# Autodesk Inventor part: Grooved Pulley2
Saved by Autodesk Inventor 2014 (Build 180170000, 170)
## iProperties
Created: 2017-06-15
Part Number: Grooved Pulley2
Material: Steel
Document SubType Name: Modeling
Designer: RMcComber
Density: 1 g/cm^3
Appearance: Steel
CustomPartVersion: 1
Author: RMcComber
Autodesk Inventor part; units mm, degrees
ref_plane "YZ Plane" through (0, 0, 0) normal (1, 0, 0) x (0, 1, 0)
ref_plane "XZ Plane" through (0, 0, 0) normal (0, 1, 0) x (-1, 0, 0)
sketch "Main Sketch" plane through (0, 0, 0) normal (1, 0, 0) x (0, 1, 0)
  line L0 (0, 19.05) -> (43.815, 19.05)
  line L1 (43.815, 19.05) -> (43.815, 15.8043)
  line L2 (43.815, 15.8043) -> (32.131, 12.2321)
  line L3 (32.131, 12.2321) -> (32.131, 6.8179)
  line L4 (32.131, 6.8179) -> (43.815, 3.2457)
  line L5 (43.815, 3.2457) -> (43.815, 0)
  line L6 (43.815, 0) -> (0, 0)
  line L7 (40.64, 14.8336) -> (40.64, 4.2164) construction
  line L8 (32.131, 9.525) -> (40.64, 9.525) construction
  line L9 (43.815, 15.8043) -> (43.815, 3.2457)
  line L10 (0, -4) -> (0, 24) projected
  line L11 (0, 0) -> (0, 19.05)
  dimension "d0" = 10.6172
  dimension "d1" = 34
  dimension "d2" = 3.175
  dimension "d6" = 19.05
  dimension "d21" = 81.28
  dimension "d25" = 11.684
  dimension "d27" = 9.525
  constraints: 22 end point, 5 perpendicular, 2 collinear, 2 midpoint, 2 point on line, 1 parallel
  measures "d0" distance of L7.start L7.end
  measures "d1" angle of L2 L4
  measures "d2" distance between parallel lines of L1 L7
  measures "d6" distance between parallel lines of L6 L0
  measures "d21" diameter of L7 L10
  measures "d25" distance between parallel lines of L3 L9
  measures "d27" distance between parallel lines of L6 L8
ref_plane "Belt Plane" through (0, 32.131, 9.525) normal (0, 0, 1) x (1, 0, 0)
revolve "Body" add sketch "Main Sketch" angle 360 about axis through (0, 0, -10) along (0, 0, 1)
revolve "Groove" cut sketch "Main Sketch" angle 360 about axis through (0, 0, -10) along (0, 0, 1) contours L9 L4 L3 L2
fillet "Fillet External" [suppressed]
fillet "Fillet Internal" [suppressed]
pattern_of_one "Groove Pattern"
equation "\"d0\" = da_Bw"
equation "\"d1\" = da_Alfa"
equation "\"d2\" = da_c"
equation "\"d21\" = da_Dw"
equation "\"d25\" = da_Hd"
equation "\"d27\" = da_Se"
equation "\"da_r1\" = 0"
equation "\"da_r2\" = 0"
equation "\"d18\" = da_Sg"
equation "\"d5\" = da_Se"
equation "\"da_Bw\" = 10.6172"
equation "\"da_Alfa\" = 34deg"
equation "\"da_c\" = 3.175"
equation "\"da_Dw\" = 81.28"
equation "\"da_Hd\" = 11.684"
equation "\"da_Se\" = 9.525"
equation "\"da_Sg\" = 15.875"
body "Solid1"
